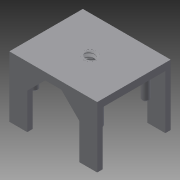
# Autodesk Inventor part: base
Saved by Autodesk Inventor 2015 (Build 190159000, 159)
## iProperties
Created: 2016-09-16
Part Number: base
Material: Generic
Document SubType Name: Modeling
Designer: spichelh
Density: 1 g/cm^3
Appearance: Default
Author: spichelh
Autodesk Inventor part; units mm, degrees
ref_plane "YZ Plane" through (0, 0, 0) normal (1, 0, 0) x (0, 1, 0)
ref_plane "XZ Plane" through (0, 0, 0) normal (0, 1, 0) x (-1, 0, 0)
ref_plane "XY Plane" through (0, 0, 0) normal (0, 0, 1) x (1, 0, 0)
sketch "Sketch1" plane through (0, 0, 0) normal (0, 1, 0) x (-1, 0, 0)
  line L0 (37.7582, 29.7546) -> (27.7582, 29.7546)
  line L1 (27.7582, 29.7546) -> (27.7582, 32.7546)
  line L2 (27.7582, 32.7546) -> (37.7582, 32.7546)
  line L3 (37.7582, 32.7546) -> (37.7582, 29.7546)
  line L4 (13.2582, 35.3764) -> (13.2582, -8.2064) construction
  line L5 (44.2482, 12.2546) -> (-17.6328, 12.2546) construction
  line L6 (-11.2418, 29.7546) -> (-1.2418, 29.7546)
  line L7 (-1.2418, 29.7546) -> (-1.2418, 32.7546)
  line L8 (-1.2418, 32.7546) -> (-11.2418, 32.7546)
  line L9 (-11.2418, 32.7546) -> (-11.2418, 29.7546)
  line L10 (37.7582, -5.2454) -> (27.7582, -5.2454)
  line L11 (27.7582, -5.2454) -> (27.7582, -8.2454)
  line L12 (27.7582, -8.2454) -> (37.7582, -8.2454)
  line L13 (37.7582, -8.2454) -> (37.7582, -5.2454)
  line L14 (-11.2418, -5.2454) -> (-1.2418, -5.2454)
  line L15 (-1.2418, -5.2454) -> (-1.2418, -8.2454)
  line L16 (-1.2418, -8.2454) -> (-11.2418, -8.2454)
  line L17 (-11.2418, -8.2454) -> (-11.2418, -5.2454)
  line L18 (36.2543, 14.0042) -> (36.5044, 14.2541) construction
  line L19 (36.5044, 14.2541) -> (36.5061, 20.9041) construction
  line L20 (36.5061, 20.9041) -> (36.2562, 21.1542) construction
  line L21 (36.2562, 21.1542) -> (32.9562, 21.155) construction
  arc A0 (32.7562, 21.3551) -> (32.9562, 21.155) centre (32.9562, 21.355) ccw construction
  line L22 (32.7562, 21.3551) -> (32.7572, 24.9551) construction
  arc A1 (32.9573, 25.155) -> (32.7572, 24.9551) centre (32.9572, 24.955) ccw construction
  line L23 (32.9573, 25.155) -> (36.2573, 25.1542) construction
  line L24 (36.2573, 25.1542) -> (36.5073, 25.4041) construction
  line L25 (36.5073, 25.4041) -> (36.5083, 28.9041) construction
  line L26 (36.5083, 28.9041) -> (-9.9917, 28.9165) construction
  line L27 (-9.9917, 28.9165) -> (-9.9927, 25.4165) construction
  line L28 (-9.9927, 25.4165) -> (-9.7427, 25.1664) construction
  line L29 (-6.4427, 25.1655) -> (-9.7427, 25.1664) construction
  arc A2 (-6.2428, 24.9655) -> (-6.4427, 25.1655) centre (-6.4428, 24.9655) ccw construction
  line L30 (-6.2438, 21.3655) -> (-6.2428, 24.9655) construction
  arc A3 (-6.4438, 21.1655) -> (-6.2438, 21.3655) centre (-6.4438, 21.3655) ccw construction
  line L31 (-9.7438, 21.1664) -> (-6.4438, 21.1655) construction
  line L32 (-9.7438, 21.1664) -> (-9.9939, 20.9165) construction
  line L33 (-9.9939, 20.9165) -> (-9.9956, 14.2665) construction
  line L34 (-9.9956, 14.2665) -> (-9.7457, 14.0164) construction
  line L35 (-8.2457, 14.016) -> (-9.7457, 14.0164) construction
  arc A4 (-8.2466, 10.516) -> (-8.2457, 14.016) centre (-8.2462, 12.266) ccw construction
  line L36 (-9.7466, 10.5164) -> (-8.2466, 10.516) construction
  line L37 (-9.7466, 10.5164) -> (-9.9967, 10.2665) construction
  line L38 (-9.9967, 10.2665) -> (-9.9985, 3.6165) construction
  line L39 (-9.9985, 3.6165) -> (-9.7485, 3.3664) construction
  line L40 (-6.4485, 3.3655) -> (-9.7485, 3.3664) construction
  arc A5 (-6.2486, 3.1655) -> (-6.4485, 3.3655) centre (-6.4486, 3.1655) ccw construction
  line L41 (-6.2496, -0.4345) -> (-6.2486, 3.1655) construction
  arc A6 (-6.4496, -0.6345) -> (-6.2496, -0.4345) centre (-6.4496, -0.4345) ccw construction
  line L42 (-9.7496, -0.6336) -> (-6.4496, -0.6345) construction
  line L43 (-9.7496, -0.6336) -> (-9.9997, -0.8835) construction
  line L44 (-9.9997, -0.8835) -> (-10.0006, -4.3835) construction
  line L45 (-10.0006, -4.3835) -> (36.4994, -4.3959) construction
  line L46 (36.4994, -4.3959) -> (36.5003, -0.8959) construction
  line L47 (36.5003, -0.8959) -> (36.2504, -0.6458) construction
  line L48 (36.2504, -0.6458) -> (32.9504, -0.645) construction
  arc A7 (32.7504, -0.4449) -> (32.9504, -0.645) centre (32.9504, -0.445) ccw construction
  line L49 (32.7504, -0.4449) -> (32.7514, 3.1551) construction
  arc A8 (32.9515, 3.355) -> (32.7514, 3.1551) centre (32.9514, 3.155) ccw construction
  line L50 (32.9515, 3.355) -> (36.2515, 3.3542) construction
  line L51 (36.2515, 3.3542) -> (36.5015, 3.6041) construction
  line L52 (36.5015, 3.6041) -> (36.5033, 10.2541) construction
  line L53 (36.5033, 10.2541) -> (36.2534, 10.5042) construction
  line L54 (36.2534, 10.5042) -> (34.7534, 10.5046) construction
  arc A9 (34.7543, 14.0046) -> (34.7534, 10.5046) centre (34.7538, 12.2546) ccw construction
  line L55 (34.7543, 14.0046) -> (36.2543, 14.0042) construction
  line L56 (-3.6005, -4.1352) -> (30.0995, -4.1442) construction
  line L57 (-3.5918, 28.6648) -> (-3.6005, -4.1352) construction
  line L58 (30.1082, 28.6558) -> (-3.5918, 28.6648) construction
  line L59 (30.0995, -4.1442) -> (30.1082, 28.6558) construction
  circle A10 centre (34.7578, 27.1546) radius 0.5 construction
  line L60 (36.2583, 29.1542) -> (36.5083, 28.9041) construction
  line L61 (-9.7417, 29.1664) -> (36.2583, 29.1542) construction
  line L62 (-9.9917, 28.9165) -> (-9.7417, 29.1664) construction
  line L63 (36.5083, 28.9041) -> (-9.9917, 28.9165) construction
  line L64 (36.7574, 25.654) -> (36.5073, 25.4041) construction
  line L65 (36.7582, 28.654) -> (36.7574, 25.654) construction
  line L66 (36.5083, 28.9041) -> (36.7582, 28.654) construction
  line L67 (36.5073, 25.4041) -> (36.5083, 28.9041) construction
  point P0 (0, 0)
  point P1 (13.2582, 28.6603)
  dimension "d0" = 3
  dimension "d1" = 10
  dimension "d4" = 0.015
  dimension "d5" = 35
  dimension "d6" = 29
  constraints: 36 end point, 12 symmetric about line, 2 horizontal, 2 parallel, 2 point on line, 1 midpoint, 1 perpendicular, 1 vertical
  measures "d0" distance of L2.end L0.start
  measures "d1" distance between parallel lines of L1 L3
  measures "d4" angle of L3 L65
  measures "d5" diameter of L0 L5
  measures "d6" distance between parallel lines of L15 L11
extrude "Extrusion1" add sketch "Sketch1" along normal blind 30
sketch "Sketch2" plane through (0, 30, 0) normal (0, 1, 0) x (1, 0, 0)
  line L0 (-37.7582, -32.7546) -> (11.2418, -32.7546)
  line L1 (11.2418, -32.7546) -> (11.2418, 8.2454)
  line L2 (11.2418, 8.2454) -> (-37.7582, 8.2454)
  line L3 (-37.7582, 8.2454) -> (-37.7582, -32.7546)
  point P0 (0, 0)
  constraints: 8 end point, 2 parallel, 1 horizontal, 1 perpendicular
extrude "Extrusion2" add sketch "Sketch2" along normal blind 4
chamfer "Chamfer1" distance 10 angle 45 4 edges at (1.2418, 30, 31.2546) (-27.7582, 30, 31.2546) (-27.7582, 30, -6.7454) (1.2418, 30, -6.7454)
sketch "Sketch3" plane through (0, 34, 0) normal (0, 1, 0) x (1, 0, 0)
  circle A0 centre (-13.2582, -12.2546) radius 4
  line L0 (11.2418, 8.2454) -> (-37.7582, -32.7546) construction
  line L1 (-37.7582, -32.7546) -> (11.2418, -32.7546) construction
  line L2 (11.2418, -32.7546) -> (11.2418, 8.2454) construction
  line L3 (11.2418, 8.2454) -> (-37.7582, 8.2454) construction
  line L4 (-37.7582, 8.2454) -> (-37.7582, -32.7546) construction
  line L5 (-37.7582, 8.2454) -> (11.2418, -32.7546) construction
  point P0 (0, 0)
  dimension "d12" = 8
  constraints: 4 end point, 2 midpoint, 1 centre point
  measures "d12" diameter of A0
extrude "Extrusion3" cut sketch "Sketch3" against normal blind 5
sketch "Sketch4" plane through (0, 30, 0) normal (0, -1, 0) x (1, 0, 0)
  circle A0 centre (-31.2582, 25.2546) radius 1.95
  circle A1 centre (-13.2582, 12.2546) radius 4 construction
  line L0 (-8.7582, -5.2454) -> (-8.7582, -8.2454) construction
  line L1 (-8.7582, -5.2454) -> (11.2418, -5.2454) construction
  line L2 (11.2418, 29.7546) -> (11.2418, -5.2454) construction
  line L3 (11.2418, 29.7546) -> (-8.7582, 29.7546) construction
  line L4 (-8.7582, 32.7546) -> (-8.7582, 29.7546) construction
  line L5 (-17.7582, 32.7546) -> (-8.7582, 32.7546) construction
  line L6 (-17.7582, 29.7546) -> (-17.7582, 32.7546) construction
  line L7 (-17.7582, 29.7546) -> (-37.7582, 29.7546) construction
  line L8 (-37.7582, -5.2454) -> (-37.7582, 29.7546) construction
  line L9 (-37.7582, -5.2454) -> (-17.7582, -5.2454) construction
  line L10 (-17.7582, -8.2454) -> (-17.7582, -5.2454) construction
  line L11 (-8.7582, -8.2454) -> (-17.7582, -8.2454) construction
  line L12 (-13.2582, 12.2546) -> (-30.8734, 12.2546) construction
  line L13 (-13.2582, 12.2546) -> (-13.2582, 27.6236) construction
  circle A2 centre (4.7418, 25.2546) radius 1.95
  circle A3 centre (-31.2582, -0.7454) radius 1.95
  circle A4 centre (4.7418, -0.7454) radius 1.95
  point P0 (0, 0)
  dimension "d15" = 3.9
  dimension "d16" = 26
  dimension "d17" = 36
  constraints: 4 centre point, 4 end point, 3 symmetric about line, 1 horizontal, 1 vertical, 3 other
  measures "d15" diameter of A0
  measures "d16" distance of A4.centre A2.centre
  measures "d17" distance of A3.centre A4.centre
extrude "Extrusion4" add sketch "Sketch4" along normal blind 15
chamfer "Chamfer2" distance 1 angle 45 4 edges at (-33.2082, 15, 25.2546) (-33.2082, 15, -0.7454) (2.7918, 15, -0.7454) (2.7918, 15, 25.2546)
thread "Thread1" size "1-12 UNF" class "2B" standard "ANSI Unified Screw Threads" full length
sketch "Sketch6" plane through (-13.2582, 30, 12.2546) normal (-1, 0, 0) x (0, 0, 1)
  line L0 (4, 0) -> (4, 4)
  line L1 (4, 4) -> (2.6187, 4)
  line L2 (2.6187, 4) -> (2.6187, 0)
  line L3 (2.6187, 0) -> (4, 0)
  line L4 (0, -36.8) -> (0, 10.8) projected
  constraints: 8 end point
revolve "Revolution1" add sketch "Sketch6" angle 360 about axis through (-13.2582, 30, 12.2546) along (0, 1, 0) separate body
sketch "Sketch5" plane through (-13.2582, 30, 16.2546) normal (1, 0, 0) x (0, 1, 0)
  line L0 (-1.2541, -0.1131) -> (-1.0584, -0.1131) construction
  line L1 (0.1955, -1.2685) -> (-0.0001, -1.6074) construction
  line L2 (-2.1168, -1.6074) -> (-2.3124, -1.2685) construction
  line L3 (-0.8628, -0.1131) -> (-1.0584, 0.2257) construction
  line L4 (-1.0584, 0.2257) -> (-1.2541, -0.1131) construction
  line L5 (-2.1168, -1.6074) -> (-1.9211, -1.2685) construction
  line L6 (-0.8628, -0.1131) -> (-0.1957, -1.2685)
  line L7 (-2.3124, -1.2685) -> (-1.9211, -1.2685) construction
  arc A0 (-2.3124, -1.2685) -> (-2.1168, -1.3815) centre (-2.1168, -1.1556) ccw construction
  line L8 (0.1955, -1.2685) -> (-0.1957, -1.2685) construction
  line L9 (-2.1168, -1.6074) -> (-2.1168, -1.2685) construction
  line L10 (-0.0001, -1.6074) -> (-0.0001, -1.2685) construction
  line L11 (-1.0584, 0.2257) -> (-1.0584, -0.0002) construction
  line L12 (-2.1168, -1.3815) -> (-0.0001, -1.3815)
  arc A1 (-2.1168, -1.3815) -> (-1.9211, -1.2685) centre (-2.1168, -1.1556) ccw
  line L13 (-0.1957, -1.2685) -> (-0.0001, -1.6074) construction
  line L14 (-1.9211, -1.2685) -> (-1.2541, -0.1131)
  line L15 (-0.0001, -0.0002) -> (-0.0001, 0.0177)
  line L16 (-0.0001, 0.0177) -> (-0.0001, -0.0002)
  line L17 (-0.0001, -0.0002) -> (0.0334, -0.0002)
  arc A2 (-0.1957, -1.2685) -> (-0.0001, -1.3815) centre (-0.0001, -1.1556) ccw
  arc A3 (-0.0001, -1.3815) -> (0.1955, -1.2685) centre (-0.0001, -1.1556) ccw construction
  arc A4 (-1.0584, -0.0002) -> (-1.2541, -0.1131) centre (-1.0584, -0.2261) ccw
  arc A5 (-0.8628, -0.1131) -> (-1.0584, -0.0002) centre (-1.0584, -0.2261) ccw
  line L18 (-1.0584, -0.0002) -> (-1.0584, -0.1131) construction
  line L19 (-1.0584, -0.1131) -> (-0.8628, -0.1131) construction
  dimension "d25" = 60
  dimension "d26" = 0.3388
  dimension "d27" = 0.3388
  dimension "Sketch5_ThreadOffset" = 0
  dimension "Sketch5_MajorRadius" = 1.3813
  dimension "d30" = 2.1167
  dimension "Sketch5_MinorRadius" = 0
  constraints: 40 end point, 12 point on circle, 10 parallel, 8 tangent, 6 centre point, 6 collinear, 2 midpoint, 2 point on line, 1 horizontal, 1 perpendicular, 3 other
  measures "d25" angle of L6 L14
  measures "d26" distance of L3.end L0.end
  measures "d27" distance of L1.end L10.end
  measures "Sketch5_ThreadOffset" distance between parallel lines of L15 L10
  measures "Sketch5_MajorRadius" distance from line of L12 L15.start
  measures "d30" distance from line of L1.end L9
  measures "Sketch5_MinorRadius" distance edge to line of A5 L17
coil "Coil1" sketch "Sketch5" operation cut axis through (-13.2582, 30, 12.2546) along (0, 1, 0) pitch 2.1188 turns 3.885878 hand right bodies 2
equation "\"d25\" = d32"
equation "\"d26\" = 0.160083 * Sketch5_Pitch"
equation "\"d27\" = 0.160083 * Sketch5_Pitch"
equation "\"d30\" = Sketch5_Pitch"
equation "\"d32\" = 60deg"
equation "\"Sketch5_Pitch\" = 2.11667"
body "Solid1"
body "Solid2"
